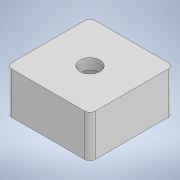
# Autodesk Inventor part: 限位開關
Saved by Autodesk Inventor 2021 (Build 250183000, 183)
## iProperties
Created: 2023-03-17
Part Number: 限位開關
Material: 一般
Document SubType Name: Modeling
Designer: brian
Density: 1 g/cm^3
Appearance: 預設
Author: brian
Autodesk Inventor part; units mm, degrees
ref_plane "YZ Plane" through (0, 0, 0) normal (1, 0, 0) x (0, 1, 0)
ref_plane "XZ Plane" through (0, 0, 0) normal (0, 1, 0) x (-1, 0, 0)
ref_plane "XY Plane" through (0, 0, 0) normal (0, 0, 1) x (1, 0, 0)
sketch "草圖2" plane through (0, 0, 0) normal (0, 1, 0) x (-1, 0, 0)
  line L0 (-15, 15) -> (15, 15)
  line L1 (15, 15) -> (15, -15)
  line L2 (15, -15) -> (-15, -15)
  line L3 (-15, -15) -> (-15, 15)
  line L4 (-15, 15) -> (15, -15) construction
  line L5 (15, 15) -> (-15, -15) construction
  line L6 (-10.1, 10.1) -> (10.1, 10.1)
  line L7 (10.1, 10.1) -> (10.1, -10.1)
  line L8 (10.1, -10.1) -> (-10.1, -10.1)
  line L9 (-10.1, -10.1) -> (-10.1, 10.1)
  line L10 (-10.1, 10.1) -> (10.1, -10.1) construction
  line L11 (10.1, 10.1) -> (-10.1, -10.1) construction
  point P0 (0, 0)
  dimension "d4" = 30
  dimension "d5" = 30
  dimension "d6" = 20.2
  dimension "d7" = 20.2
  constraints: 24 end point, 4 midpoint, 4 parallel, 2 horizontal, 2 perpendicular
  measures "d4" distance of L1.end L2.end
  measures "d5" distance of L0.end L1.end
  measures "d6" distance of L7.end L8.end
  measures "d7" distance of L6.end L7.end
extrude "擠出2" add sketch "草圖2" along normal blind 15
sketch "草圖3" plane through (0, 15, 0) normal (0, 1, 0) x (1, 0, 0)
  line L0 (15, 15) -> (-15, 15) projected
  line L1 (-15, 15) -> (-15, -15) projected
  line L2 (-15, -15) -> (15, -15) projected
  line L3 (15, -15) -> (15, 15) projected
  line L4 (10.1, -10.1) -> (-10.1, -10.1) projected
  line L5 (-10.1, -10.1) -> (-10.1, 10.1) projected
  line L6 (-10.1, 10.1) -> (10.1, 10.1) projected
  line L7 (10.1, 10.1) -> (10.1, -10.1) projected
  point P0 (0, 0)
extrude "擠出3" add sketch "草圖3" against normal blind 8 contours L4 L5 L6 L7
sketch "草圖4" plane through (0, 15, 0) normal (0, 1, 0) x (1, 0, 0)
  circle A0 centre (0, 0) radius 2.1
  dimension "d12" = 4.2
  constraints: 1 centre point, 1 coincident
  measures "d12" diameter of A0
hole "孔1" at (0, 15, 0) direction (0, -1, 0) diameter 4.2 end through all counterbore diameter 7.2 counterbore depth 4
sketch "草圖5" plane through (-15, 0, -15) normal (-1, 0, 0) x (0, 0, 1)
  line L0 (10.25, 7) -> (19.75, 7) construction
  line L1 (0, 0) -> (30, 0) construction
  line L2 (0, 15) -> (30, 15) construction
  point P0 (15, 0)
  point P1 (15, 7)
  point P2 (15, 0)
  dimension "d20" = 9.5
  dimension "d21" = 8
  constraints: 2 end point, 2 midpoint, 1 horizontal, 1 vertical alignment
  measures "d20" distance of L0.end L0.start
  measures "d21" distance between parallel lines of L2 L0
hole "孔2" at (-15, 7, -4.75) at (-15, 7, 4.75) direction (1, 0, 0) diameter 2 depth 4.9
fillet "圓角1" radius 2 4 edges at (-15, 7.5, -15) (-15, 7.5, 15) (15, 7.5, -15) (15, 7.5, 15)
sketch "草圖1" plane through (0, 0, 0) normal (0, 1, 0) x (-1, 0, 0)
  line L0 (-10, 10) -> (10, 10)
  line L1 (10, 10) -> (10, -10)
  line L2 (10, -10) -> (-10, -10)
  line L3 (-10, -10) -> (-10, 10)
  line L4 (-10, 10) -> (10, -10) construction
  line L5 (10, 10) -> (-10, -10) construction
  point P0 (0, 0)
  dimension "d2" = 20
  dimension "d3" = 20
  constraints: 12 end point, 2 midpoint, 2 parallel, 1 horizontal, 1 perpendicular
  measures "d2" distance of L1.end L2.end
  measures "d3" distance of L0.end L1.end
equation "\"d6\" = d7"
